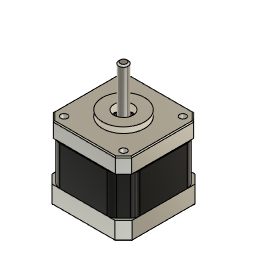
eixo Z 1 v26 (Autodesk Fusion 360 archive; units mm, degrees)
design "motor-17hs4401"
Autodesk Fusion 360 part; units mm, degrees
sketch "Sketch1" plane through (0, 0, 0) normal (0, 0, 1) x (1, 0, 0)
  line L0 (4.1049, 0.5798) -> (36.8951, 0.5798)
  line L1 (41.425, 5.1097) -> (41.425, 37.8999)
  line L2 (36.8951, 42.4298) -> (4.1049, 42.4298)
  line L3 (-0.425, 37.8999) -> (-0.425, 5.1097)
  line L4 (-0.425, 37.8999) -> (4.1049, 42.4298)
  line L5 (36.8951, 0.5798) -> (41.425, 5.1097)
  line L6 (-0.425, 5.1097) -> (4.1049, 0.5798)
  line L7 (36.8951, 42.4298) -> (41.425, 37.8999)
  circle A0 centre (20.5, 21.5048) radius 4.425
  circle A1 centre (5, 37.0048) radius 3.1
  line L8 (-0.425, 21.5048) -> (41.425, 21.5048) construction
  line L9 (20.5, 42.4298) -> (20.5, 0.5798) construction
  line L10 (5, 37.0048) -> (36, 37.0048) construction
  line L11 (36, 37.0048) -> (36, 6.0048) construction
  line L12 (36, 6.0048) -> (5, 6.0048) construction
  line L13 (5, 6.0048) -> (5, 37.0048) construction
  circle A2 centre (36, 37.0048) radius 3.1
  circle A3 centre (36, 6.0048) radius 3.1
  circle A4 centre (5, 6.0048) radius 3.1
  dimension "d3" = 45
  dimension "d4" = 45
  dimension "d5" = 41.85
  dimension "d6" = 41.85
  dimension "d7" = 52.7786
  dimension "d8" = 8.85
  dimension "d9" = 6.2
  dimension "d11" = 31
  dimension "d12" = 31
  constraint horizontal L0
  constraint vertical L1
  constraint horizontal L2
  constraint vertical L3
  constraint parallel L4 L5
  constraint equal L4 L5
  constraint parallel L6 L7
  constraint equal L0 L2
  constraint equal L4 L6
  constraint midpoint L3 L8.start
  constraint midpoint L1 L8.end
  constraint midpoint L2 L9.start
  constraint midpoint L0 L9.end
  constraint coincident A0.centre L9
  constraint coincident A0.centre L8
  constraint horizontal L10
  constraint vertical L11
  constraint horizontal L12
  constraint vertical L13
  constraint coincident A1.centre L10.start
  constraint coincident L10.end L11.start
  constraint coincident L11.end L12.start
  constraint coincident L12.end L13.start
  constraint equal A3 A4
  constraint equal A2 A3
  constraint equal A1 A2
  constraint symmetric L8 L10 L12
  measures "d3" angle of L3 L4
  measures "d4" angle of L0 L6
  measures "d5" distance of L0 L2
  measures "d6" distance of L1 L3
  measures "d7" distance of L4 L5
  measures "d8" diameter of A0
  measures "d9" diameter of A1
  measures "d11" distance of L10.end L11.end
  measures "d12" distance of L11.end L12.end
extrude "Extrude1" add sketch "Sketch1" along normal blind 9.4 makes body 1
fillet "Fillet1" radius 0.5 8 edges at (20.5, 42.4298, 0) (39.1601, 40.1649, 0) (41.425, 21.5048, 0) (39.1601, 2.8448, 0) (20.5, 0.5798, 0) (1.8399, 2.8448, 0) (1.8399, 40.1649, 0) (-0.425, 21.5048, 0) on bodies 1
sketch "Sketch2" plane through (0, 0, 9.4) normal (0, 0, 1) x (-1, 0, 0)
  circle A0 centre (-20.5, -21.5048) radius 4.425
  circle A1 centre (-36, -37.0048) radius 3.1
  circle A2 centre (-5, -37.0048) radius 3.1
  circle A3 centre (-5, -6.0048) radius 3.1
  circle A4 centre (-36, -6.0048) radius 3.1
  line L0 (0.425, -37.8999) -> (0.425, -5.1097)
  line L1 (0.425, -5.1097) -> (-4.1049, -0.5798)
  line L2 (-4.1049, -0.5798) -> (-36.8951, -0.5798)
  line L3 (-36.8951, -0.5798) -> (-41.425, -5.1097)
  line L4 (-41.425, -5.1097) -> (-41.425, -37.8999)
  line L5 (-41.425, -37.8999) -> (-36.8951, -42.4298)
  line L6 (-36.8951, -42.4298) -> (-4.1049, -42.4298)
  line L7 (-4.1049, -42.4298) -> (0.425, -37.8999)
  circle A5 centre (-20.5, -21.5048) radius 3.75
  circle A6 centre (-20.5, -21.5048) radius 2.25
  dimension "d17" = 7.5
  dimension "d18" = -1.5
  constraint concentric A0 A5
  measures "d17" diameter of A5
extrude "Extrude2" add sketch "Sketch2" against normal blind 3 separate body contours A5 makes body 2
extrude "Extrude3" add sketch "Sketch2" against normal blind 4 contours A6 bodies 2
chamfer "Chamfer1" distance 0.5 angle 45 1 edges at (22.5977, 20.6912, 5.4) on bodies 2
sketch "Sketch3" plane through (0, 0, 9.4) normal (0, 0, 1) x (-1, 0, 0)
  circle A0 centre (-20.5, -21.5048) radius 4.425
  circle A1 centre (-36, -37.0048) radius 3.1
  circle A2 centre (-5, -37.0048) radius 3.1
  circle A3 centre (-5, -6.0048) radius 3.1
  circle A4 centre (-36, -6.0048) radius 3.1
  line L0 (0.425, -37.8999) -> (0.425, -5.1097)
  line L1 (0.425, -5.1097) -> (-4.1049, -0.5798)
  line L2 (-4.1049, -0.5798) -> (-36.8951, -0.5798)
  line L3 (-36.8951, -0.5798) -> (-41.425, -5.1097)
  line L4 (-41.425, -5.1097) -> (-41.425, -37.8999)
  line L5 (-41.425, -37.8999) -> (-36.8951, -42.4298)
  line L6 (-36.8951, -42.4298) -> (-4.1049, -42.4298)
  line L7 (-4.1049, -42.4298) -> (0.425, -37.8999)
  line L8 (-8.4787, -31.5261) -> (-8.4787, -11.4835)
  line L9 (-10.4787, -9.4835) -> (-30.5213, -9.4835)
  line L10 (-32.5213, -11.4835) -> (-32.5213, -31.5261)
  line L11 (-30.5213, -33.5261) -> (-10.4787, -33.5261)
  line L12 (-10.4787, -33.5261) -> (-8.4787, -31.5261)
  line L13 (-8.4787, -11.4835) -> (-10.4787, -9.4835)
  line L14 (-30.5213, -9.4835) -> (-32.5213, -11.4835)
  line L15 (-32.5213, -31.5261) -> (-30.5213, -33.5261)
  point P0 (-8.4787, -33.5261)
  point P1 (-8.4787, -9.4835)
  point P2 (-32.5213, -9.4835)
  point P3 (-32.5213, -33.5261)
  dimension "d25" = 2
  dimension "d26" = 2
  dimension "d27" = 2
  dimension "d28" = 2
  dimension "d29" = 2
  dimension "d30" = 2
  dimension "d31" = 2
  dimension "d32" = 2
  constraint parallel L0 L8
  constraint parallel L2 L9
  constraint parallel L4 L10
  constraint parallel L6 L11
  constraint coincident L11 P0
  constraint coincident L8 P0
  constraint coincident L8 P1
  constraint coincident L9 P1
  constraint coincident L9 P2
  constraint coincident L10 P2
  constraint coincident L10 P3
  constraint coincident L11 P3
  measures "d25" distance of L11.end P0
  measures "d26" distance of L8.start P0
  measures "d27" distance of L8.end P1
  measures "d28" distance of L9.start P1
  measures "d29" distance of L9.end P2
  measures "d30" distance of L10.start P2
  measures "d31" distance of L10.end P3
  measures "d32" distance of L11.start P3
extrude "Extrude4" cut sketch "Sketch3" against normal blind 6 contours L8 L9 L10 L11 L12 L13 L14 L15 bodies 1
sketch "Sketch4" plane through (0, 0, 9.4) normal (0, 0, 1) x (-1, 0, 0)
  circle A0 centre (-20.5, -21.5048) radius 3.75
  circle A1 centre (-20.5, -21.5048) radius 6.5
  circle A2 centre (-20.5, -21.5048) radius 3.9
  dimension "d35" = 13
  dimension "d36" = -2.6
  constraint concentric A0 A1
  measures "d35" diameter of A1
extrude "Extrude5" add sketch "Sketch4" against normal blind 3 separate body contours A1 makes body 3
extrude "Extrude6" add sketch "Sketch2" against normal blind 5.5 contours A1 | A2 | A3 | A4 bodies 1
sketch "Sketch5" plane through (0, 0, 3.9) normal (0, 0, -1) x (1, 0, 0)
  circle A0 centre (36, -6.0048) radius 3.1
  circle A1 centre (36, -6.0048) radius 2.5
  arc A2 (36.5, -4.5048) -> (35.5, -4.5048) centre (36, -4.5048) ccw
  arc A3 (35.5, -7.5048) -> (36.5, -7.5048) centre (36, -7.5048) ccw
  line L0 (36, -7.5048) -> (36, -4.5048) construction
  arc A4 (37.5, -6.5048) -> (37.5, -5.5048) centre (37.5, -6.0048) ccw
  arc A5 (34.5, -5.5048) -> (34.5, -6.5048) centre (34.5, -6.0048) ccw
  line L1 (34.5, -6.0048) -> (37.5, -6.0048) construction
  line L2 (37.5, -5.5048) -> (36.5, -5.5048)
  line L3 (35.5, -5.5048) -> (34.5, -5.5048)
  line L4 (35.5, -4.5048) -> (35.5, -5.5048)
  line L5 (35.5, -6.5048) -> (35.5, -7.5048)
  line L6 (34.5, -6.5048) -> (35.5, -6.5048)
  line L7 (36.5, -6.5048) -> (37.5, -6.5048)
  line L8 (36.5, -7.5048) -> (36.5, -6.5048)
  line L9 (36.5, -5.5048) -> (36.5, -4.5048)
  circle A6 centre (5, -6.0048) radius 2.5
  line L10 (5.5, -5.5048) -> (5.5, -4.5048)
  line L11 (4.5, -4.5048) -> (4.5, -5.5048)
  arc A7 (5.5, -4.5048) -> (4.5, -4.5048) centre (5, -4.5048) ccw
  line L12 (4.5, -5.5048) -> (3.5, -5.5048)
  arc A8 (3.5, -5.5048) -> (3.5, -6.5048) centre (3.5, -6.0048) ccw
  line L13 (3.5, -6.5048) -> (4.5, -6.5048)
  line L14 (4.5, -6.5048) -> (4.5, -7.5048)
  arc A9 (4.5, -7.5048) -> (5.5, -7.5048) centre (5, -7.5048) ccw
  line L15 (5.5, -7.5048) -> (5.5, -6.5048)
  line L16 (5.5, -6.5048) -> (6.5, -6.5048)
  arc A10 (6.5, -6.5048) -> (6.5, -5.5048) centre (6.5, -6.0048) ccw
  line L17 (6.5, -5.5048) -> (5.5, -5.5048)
  circle A11 centre (36, -37.0048) radius 2.5
  line L18 (36.5, -36.5048) -> (36.5, -35.5048)
  line L19 (35.5, -35.5048) -> (35.5, -36.5048)
  arc A12 (36.5, -35.5048) -> (35.5, -35.5048) centre (36, -35.5048) ccw
  line L20 (35.5, -36.5048) -> (34.5, -36.5048)
  arc A13 (34.5, -36.5048) -> (34.5, -37.5048) centre (34.5, -37.0048) ccw
  line L21 (34.5, -37.5048) -> (35.5, -37.5048)
  line L22 (35.5, -37.5048) -> (35.5, -38.5048)
  arc A14 (35.5, -38.5048) -> (36.5, -38.5048) centre (36, -38.5048) ccw
  line L23 (36.5, -38.5048) -> (36.5, -37.5048)
  line L24 (36.5, -37.5048) -> (37.5, -37.5048)
  arc A15 (37.5, -37.5048) -> (37.5, -36.5048) centre (37.5, -37.0048) ccw
  line L25 (37.5, -36.5048) -> (36.5, -36.5048)
  circle A16 centre (5, -37.0048) radius 2.5
  line L26 (5.5, -36.5048) -> (5.5, -35.5048)
  line L27 (4.5, -35.5048) -> (4.5, -36.5048)
  arc A17 (5.5, -35.5048) -> (4.5, -35.5048) centre (5, -35.5048) ccw
  line L28 (4.5, -36.5048) -> (3.5, -36.5048)
  arc A18 (3.5, -36.5048) -> (3.5, -37.5048) centre (3.5, -37.0048) ccw
  line L29 (3.5, -37.5048) -> (4.5, -37.5048)
  line L30 (4.5, -37.5048) -> (4.5, -38.5048)
  arc A19 (4.5, -38.5048) -> (5.5, -38.5048) centre (5, -38.5048) ccw
  line L31 (5.5, -38.5048) -> (5.5, -37.5048)
  line L32 (5.5, -37.5048) -> (6.5, -37.5048)
  arc A20 (6.5, -37.5048) -> (6.5, -36.5048) centre (6.5, -37.0048) ccw
  line L33 (6.5, -36.5048) -> (5.5, -36.5048)
  point P0 (36, -6.0048)
  point P1 (36, -6.0048)
  dimension "d41" = 5
  dimension "d42" = 1
  dimension "d43" = 1
  dimension "d44" = 3
  dimension "d45" = 3
  dimension "d48" = -31
  dimension "d49" = -31
  constraint concentric A0 A1
  constraint tangent A2 L8
  constraint tangent A2 L4
  constraint parallel L4 L8
  constraint tangent A3 L4
  constraint tangent A3 L8
  constraint vertical L0
  constraint coincident P1 P0
  constraint midpoint L0 P1
  constraint tangent A4 L6
  constraint tangent A4 L2
  constraint parallel L2 L6
  constraint tangent A5 L2
  constraint tangent A5 L6
  constraint perpendicular L0 L1
  constraint midpoint L1 P1
  constraint collinear L2 L3
  constraint collinear L4 L5
  constraint collinear L6 L7
  constraint collinear L8 L9
  measures "d41" diameter of A1
  measures "d42" distance of L2 L6
  measures "d43" distance of L4 L8
  measures "d44" distance of A3.centre A2.centre
  measures "d45" distance of A5.centre A4.centre
extrude "Extrude7" add sketch "Sketch5" along normal blind 3.6 contours A1 | A6 | A11 | A16 bodies 1
fillet "Fillet2" radius 1 1 edges at (33.6692, 6.9089, 0.3) on bodies 1
fillet "Fillet3" radius 1 1 edges at (2.6692, 6.9089, 0.3) on bodies 1
fillet "Fillet4" radius 1 2 edges at (33.6692, 37.9089, 0.3) (2.6692, 37.9089, 0.3) on bodies 1
sketch "Sketch6" plane through (0, 0, 0) normal (0, 0, -1) x (1, 0, 0)
  circle A0 centre (36, -6.0048) radius 3.1
  circle A1 centre (5, -6.0048) radius 3.1
  circle A2 centre (5, -37.0048) radius 3.1
  circle A3 centre (36, -37.0048) radius 3.1
  circle A4 centre (20.5, -21.5048) radius 4.425
  line L0 (0.075, -5.3168) -> (0.075, -37.6928)
  line L1 (0.075, -37.6928) -> (4.312, -41.9298)
  line L2 (4.312, -41.9298) -> (36.688, -41.9298)
  line L3 (36.688, -41.9298) -> (40.925, -37.6928)
  line L4 (40.925, -37.6928) -> (40.925, -5.3168)
  line L5 (40.925, -5.3168) -> (36.688, -1.0798)
  line L6 (36.688, -1.0798) -> (4.312, -1.0798)
  line L7 (4.312, -1.0798) -> (0.075, -5.3168)
  line L8 (12.25, -41.9298) -> (28.75, -41.9298)
  line L9 (28.75, -41.9298) -> (28.75, -46.5798)
  line L10 (28.75, -46.5798) -> (12.25, -46.5798)
  line L11 (12.25, -46.5798) -> (12.25, -41.9298)
  line L12 (20.5, -21.5048) -> (20.5, -41.9298) construction
  line L13 (36.8951, -0.5798) -> (4.1049, -0.5798)
  dimension "d58" = 16.5
  dimension "d59" = 46
  constraint horizontal L8
  constraint vertical L9
  constraint horizontal L10
  constraint vertical L11
  constraint coincident L2 L8.start
  constraint coincident A4.centre L12.start
  constraint midpoint L2 L12.end
  constraint symmetric L8.start L8.end L12
  measures "d58" distance of L9.end L10.end
  measures "d59" distance of L10 L13
extrude "Extrude8" add sketch "Sketch6" against normal blind 2.8 contours L2 L8 L9 L10 L11 bodies 1
fillet "Fillet5" radius 0.5 3 edges at (12.25, 44.2548, 0) (20.5, 46.5798, 0) (28.75, 44.2548, 0) on bodies 1
sketch "Sketch7" plane through (0, 42.4298, 0) normal (0, 1, 0) x (-1, 0, 0)
  line L0 (-12.25, 2.8) -> (-12.25, 0.5)
  line L1 (-12.25, 0.5) -> (-4.1049, 0.5)
  line L2 (-4.1049, 0.5) -> (-4.1049, 9.4)
  line L3 (-4.1049, 9.4) -> (-36.8951, 9.4)
  line L4 (-36.8951, 9.4) -> (-36.8951, 0.5)
  line L5 (-36.8951, 0.5) -> (-28.75, 0.5)
  line L6 (-28.75, 0.5) -> (-28.75, 2.8)
  line L7 (-28.75, 2.8) -> (-12.25, 2.8)
  line L8 (-28.75, 2.8) -> (-12.25, 2.8)
  line L9 (-12.25, 2.8) -> (-12.25, 9.4)
  line L10 (-12.25, 9.4) -> (-28.75, 9.4)
  line L11 (-28.75, 9.4) -> (-28.75, 2.8)
  line L12 (-12.25, 0.5) -> (-12.25, 2.8)
  constraint horizontal L8
  constraint vertical L9
  constraint horizontal L10
  constraint vertical L11
  constraint coincident L3 L9.end
  constraint coincident L6.end L7.start
  constraint collinear L9 L12
extrude "Extrude9" cut sketch "Sketch7" against normal blind 9 contours L3 L7 L8 L9 L10 L11 bodies 1
sketch "Sketch8" plane through (0, 0, 2.8) normal (0, 0, 1) x (-1, 0, 0)
  line L0 (-28.75, -42.4298) -> (-28.75, -46.5798)
  line L1 (-28.75, -46.5798) -> (-12.25, -46.5798)
  line L2 (-12.25, -46.5798) -> (-12.25, -42.4298)
  line L3 (-12.25, -42.4298) -> (-12.25, -33.4298)
  line L4 (-12.25, -33.4298) -> (-28.75, -33.4298)
  line L5 (-28.75, -33.4298) -> (-28.75, -42.4298)
  line L6 (-13.55, -45.5798) -> (-27.45, -45.5798)
  line L7 (-27.45, -45.5798) -> (-27.45, -33.4298)
  line L8 (-27.45, -33.4298) -> (-13.55, -33.4298)
  line L9 (-13.55, -33.4298) -> (-13.55, -45.5798)
  dimension "d66" = 1.3
  dimension "d67" = 1.3
  dimension "d68" = 1
  constraint horizontal L6
  constraint vertical L7
  constraint horizontal L8
  constraint vertical L9
  constraint coincident L4 L7.end
  measures "d66" distance of L2 L9
  measures "d67" distance of L0 L7
  measures "d68" distance of L1 L6
extrude "Extrude10" add sketch "Sketch8" along normal blind 1 contours L4 L6 L7 L8 L9 bodies 1
sketch "Sketch9" plane through (0, 0, 3.8) normal (0, 0, 1) x (-1, 0, 0)
  line L0 (-13.55, -33.4298) -> (-27.45, -33.4298)
  line L1 (-27.45, -33.4298) -> (-27.45, -45.5798)
  line L2 (-27.45, -45.5798) -> (-13.55, -45.5798) construction
  line L3 (-13.55, -45.5798) -> (-13.55, -33.4298) construction
  line L4 (-12.9, -33.4298) -> (-28.1, -33.4298)
  line L5 (-28.1, -33.4298) -> (-28.1, -45.3421)
  line L6 (-28.1, -45.3421) -> (-12.9, -45.3421)
  line L7 (-12.9, -45.3421) -> (-12.9, -33.4298)
  line L8 (-28.75, -42.4298) -> (-28.75, -46.5798)
  line L9 (-12.9, -45.3421) -> (-12.25, -45.3421) construction
  line L10 (-28.1, -45.3421) -> (-28.75, -45.3421) construction
  line L11 (-12.25, -46.5798) -> (-12.25, -42.4298)
  line L12 (-13.6, -45.3421) -> (-13.6, -34.1298)
  line L13 (-13.6, -34.1298) -> (-27.4, -34.1298)
  line L14 (-27.4, -34.1298) -> (-27.4, -45.3421)
  dimension "d71" = 15.2
  dimension "d75" = -0.7
  constraint horizontal L4
  constraint vertical L5
  constraint horizontal L6
  constraint vertical L7
  constraint perpendicular L7 L9
  constraint coincident L8 L10.end
  constraint perpendicular L8 L10
  constraint coincident L9.end L11
  constraint equal L9 L10
  constraint collinear L0 L4
  measures "d71" distance of L5 L7
extrude "Extrude12" add sketch "Sketch9" along normal blind 5.5 contours L0 L1 L4 L6 L7 L12 L13 L14 | L1 L4 L5 L6 bodies 1
extrude "Extrude13" add sketch "Sketch9" along normal blind 1 contours L6 L12 L13 L14 bodies 1
sketch "Sketch10" plane through (0, 34.1298, 0) normal (0, 1, 0) x (-1, 0, 0)
  line L0 (-27.4, 4.8) -> (-13.6, 4.8)
  line L1 (-13.6, 4.8) -> (-13.6, 9.3)
  line L2 (-13.6, 9.3) -> (-27.4, 9.3)
  line L3 (-27.4, 9.3) -> (-27.4, 4.8)
  line L4 (-27, 9.3) -> (-14, 9.3)
  line L5 (-14, 9.3) -> (-14, 5)
  line L6 (-14, 5) -> (-27, 5)
  line L7 (-27, 5) -> (-27, 9.3)
  line L8 (-27.4, 4.8) -> (-27.4, 9.3)
  line L9 (-13.6, 4.8) -> (-13.6, 9.3)
  line L10 (-15, 9.3) -> (-15, 6)
  line L11 (-15, 6) -> (-26, 6)
  line L12 (-26, 6) -> (-26, 9.3)
  line L13 (-25, 8) -> (-24, 8)
  line L14 (-24, 8) -> (-24, 7)
  line L15 (-24, 7) -> (-25, 7)
  line L16 (-25, 7) -> (-25, 8)
  line L17 (-22.4, 8) -> (-22.4, 7)
  line L18 (-23.4, 8) -> (-22.4, 8)
  line L19 (-23.4, 7) -> (-23.4, 8)
  line L20 (-22.4, 7) -> (-23.4, 7)
  line L21 (-20.8, 8) -> (-20.8, 7)
  line L22 (-21.8, 8) -> (-20.8, 8)
  line L23 (-21.8, 7) -> (-21.8, 8)
  line L24 (-20.8, 7) -> (-21.8, 7)
  line L25 (-19.2, 8) -> (-19.2, 7)
  line L26 (-20.2, 8) -> (-19.2, 8)
  line L27 (-20.2, 7) -> (-20.2, 8)
  line L28 (-19.2, 7) -> (-20.2, 7)
  line L29 (-17.6, 8) -> (-17.6, 7)
  line L30 (-18.6, 8) -> (-17.6, 8)
  line L31 (-18.6, 7) -> (-18.6, 8)
  line L32 (-17.6, 7) -> (-18.6, 7)
  line L33 (-16, 8) -> (-16, 7)
  line L34 (-17, 8) -> (-16, 8)
  line L35 (-17, 7) -> (-17, 8)
  line L36 (-16, 7) -> (-17, 7)
  dimension "d82" = 0.4
  dimension "d83" = 0.4
  dimension "d85" = 0.2
  dimension "d87" = 1
  dimension "d88" = 1
  dimension "d89" = 1
  dimension "d90" = 1
  dimension "d91" = 1
  dimension "d92" = 1
  dimension "d93" = 1
  dimension "d96" = 8
  dimension "d97" = 0
  constraint horizontal L4
  constraint vertical L5
  constraint horizontal L6
  constraint vertical L7
  constraint collinear L2 L4
  constraint parallel L5 L10
  constraint parallel L6 L11
  constraint parallel L7 L12
  constraint coincident L4 L12.end
  constraint coincident L4 L10.start
  constraint horizontal L13
  constraint vertical L14
  constraint horizontal L15
  constraint vertical L16
  measures "d82" distance of L7 L8
  measures "d83" distance of L5 L9
  measures "d85" distance of L0 L6
  measures "d87" distance of L7 L12
  measures "d88" distance of L5 L10
  measures "d89" distance of L6 L11
  measures "d90" distance of L13.start L13.end
  measures "d91" distance of L13.end L14.end
  measures "d92" distance of L12 L16
  measures "d93" distance of L11 L15
extrude "Extrude14" add sketch "Sketch10" along normal blind 13 contours L2 L4 L5 L6 L7 L10 L11 L12 bodies 1
extrude "Extrude15" add sketch "Sketch10" along normal blind 12 contours L13 L14 L15 L16 | L17 L18 L19 L20 | L21 L22 L23 L24 | L25 L26 L27 L28 | L29 L30 L31 L32 | L33 L34 L35 L36 bodies 1
sketch "Sketch11" plane through (0, 0, 9.4) normal (0, 0, 1) x (-1, 0, 0)
  line L0 (-28.75, -42.4298) -> (-28.75, -33.5261)
  line L1 (-28.75, -33.5261) -> (-30.5213, -33.5261)
  line L2 (-30.5213, -33.5261) -> (-32.5213, -31.5261)
  line L3 (-32.5213, -31.5261) -> (-32.5213, -11.4835)
  line L4 (-32.5213, -11.4835) -> (-30.5213, -9.4835)
  line L5 (-30.5213, -9.4835) -> (-10.4787, -9.4835)
  line L6 (-10.4787, -9.4835) -> (-8.4787, -11.4835)
  line L7 (-8.4787, -11.4835) -> (-8.4787, -31.5261)
  line L8 (-8.4787, -31.5261) -> (-10.4787, -33.5261)
  line L9 (-10.4787, -33.5261) -> (-12.25, -33.5261)
  line L10 (-12.25, -33.5261) -> (-12.25, -42.4298)
  line L11 (-12.25, -42.4298) -> (-4.1049, -42.4298)
  line L12 (-4.1049, -42.4298) -> (0.425, -37.8999)
  line L13 (0.425, -37.8999) -> (0.425, -5.1097)
  line L14 (0.425, -5.1097) -> (-4.1049, -0.5798)
  line L15 (-4.1049, -0.5798) -> (-36.8951, -0.5798)
  line L16 (-36.8951, -0.5798) -> (-41.425, -5.1097)
  line L17 (-41.425, -5.1097) -> (-41.425, -37.8999)
  line L18 (-41.425, -37.8999) -> (-36.8951, -42.4298)
  line L19 (-36.8951, -42.4298) -> (-28.75, -42.4298)
  line L20 (-8.1461, -42.4298) -> (-32.8539, -42.4298)
  line L21 (-41.425, -33.8587) -> (-41.425, -9.1509)
  line L22 (-32.8539, -0.5798) -> (-8.1461, -0.5798)
  line L23 (0.425, -7.0798) -> (0.425, -33.8587)
  line L24 (-4.6105, -40.9654) -> (-1.0395, -37.3943)
  line L25 (-4.6105, -2.0443) -> (0.425, -7.0798)
  line L26 (-36.3895, -2.0443) -> (-39.9605, -5.6154)
  line L27 (-36.3895, -40.9654) -> (-39.9605, -37.3943)
  arc A0 (-1.0395, -37.3943) -> (0.425, -33.8587) centre (-4.575, -33.8587) ccw
  arc A1 (-8.1461, -42.4298) -> (-4.6105, -40.9654) centre (-8.1461, -37.4298) ccw
  arc A2 (-36.3895, -40.9654) -> (-32.8539, -42.4298) centre (-32.8539, -37.4298) ccw
  arc A3 (-41.425, -33.8587) -> (-39.9605, -37.3943) centre (-36.425, -33.8587) ccw
  arc A4 (-39.9605, -5.6154) -> (-41.425, -9.1509) centre (-36.425, -9.1509) ccw
  arc A5 (-32.8539, -0.5798) -> (-36.3895, -2.0443) centre (-32.8539, -5.5798) ccw
  arc A6 (-4.6105, -2.0443) -> (-8.1461, -0.5798) centre (-8.1461, -5.5798) ccw
  point P0 (-6.075, -42.4298)
  point P1 (0.425, -35.9298)
  point P2 (0.425, -42.4298)
  point P3 (-6.075, -0.5798)
  point P4 (0.425, -0.5798)
  point P5 (-34.925, -0.5798)
  point P6 (-41.425, -7.0798)
  point P7 (-41.425, -0.5798)
  point P8 (-34.925, -42.4298)
  point P9 (-41.425, -35.9298)
  point P10 (-41.425, -42.4298)
  dimension "d102" = 6.5
  dimension "d103" = 6.5
  dimension "d104" = 6.5
  dimension "d105" = 6.5
  dimension "d106" = 6.5
  dimension "d107" = 6.5
  dimension "d108" = 6.5
  dimension "d109" = 6.5
  dimension "d110" = 5
  constraint horizontal L20
  constraint vertical L21
  constraint horizontal L22
  constraint vertical L23
  constraint collinear L17 L21
  constraint collinear L15 L22
  constraint collinear L13 L23
  constraint collinear L19 L20
  constraint coincident L20 P2
  constraint coincident L23 P2
  constraint coincident L22 P4
  constraint coincident L23 P4
  constraint coincident L22 P7
  constraint coincident L21 P7
  constraint coincident L20 P10
  constraint coincident L21 P10
  constraint coincident P1 L24
  constraint coincident L23 P1
  constraint tangent L24 A0
  constraint tangent L23 A0
  constraint coincident P0 L24
  constraint coincident L20 P0
  constraint tangent L24 A1
  constraint tangent L20 A1
  constraint equal A0 A1
  constraint coincident L20 P8
  constraint coincident P8 L27
  constraint tangent L20 A2
  constraint tangent L27 A2
  constraint equal A0 A2
  constraint coincident P9 L27
  constraint coincident L21 P9
  constraint tangent L27 A3
  constraint tangent L21 A3
  constraint equal A0 A3
  constraint coincident P6 L26
  constraint coincident L21 P6
  constraint tangent L26 A4
  constraint tangent L21 A4
  constraint equal A0 A4
  constraint coincident L22 P5
  constraint coincident P5 L26
  constraint tangent L22 A5
  constraint tangent L26 A5
  constraint equal A0 A5
  constraint coincident P3 L25
  constraint coincident L22 P3
  constraint tangent L25 A6
  constraint tangent L22 A6
  constraint equal A0 A6
  measures "d102" distance of P0 P2
  measures "d103" distance of P1 P2
  measures "d104" distance of P3 P4
  measures "d105" distance of L23.start P4
  measures "d106" distance of P5 P7
  measures "d107" distance of P6 P7
  measures "d108" distance of P8 P10
  measures "d109" distance of P9 P10
  measures "d110" radius of A0
extrude "Extrude16" add sketch "Sketch11" along normal blind 20.5 separate body contours L0 L1 L2 L3 L4 L5 L6 L7 L8 L9 L10 L11 L13 L15 L17 L19 L20 L21 L22 L23 L24 L25 L26 L27 A0 A1 A2 A3 A4 A5 A6 | L0 L1 L2 L3 L4 L5 L6 L7 L8 L9 L10 L20 makes body 4
sketch "Sketch12" plane through (0, 0, 29.9) normal (0, 0, 1) x (-1, 0, 0)
  line L0 (0.425, -7.0798) -> (-4.6105, -2.0443)
  arc A0 (-4.6105, -2.0443) -> (-8.1461, -0.5798) centre (-8.1461, -5.5798) ccw
  line L1 (-8.1461, -0.5798) -> (-32.8539, -0.5798)
  arc A1 (-32.8539, -0.5798) -> (-36.3895, -2.0443) centre (-32.8539, -5.5798) ccw
  line L2 (-36.3895, -2.0443) -> (-39.9605, -5.6154)
  arc A2 (-39.9605, -5.6154) -> (-41.425, -9.1509) centre (-36.425, -9.1509) ccw
  line L3 (-41.425, -9.1509) -> (-41.425, -33.8587)
  arc A3 (-41.425, -33.8587) -> (-39.9605, -37.3943) centre (-36.425, -33.8587) ccw
  line L4 (-39.9605, -37.3943) -> (-36.3895, -40.9654)
  arc A4 (-36.3895, -40.9654) -> (-32.8539, -42.4298) centre (-32.8539, -37.4298) ccw
  line L5 (-32.8539, -42.4298) -> (-8.1461, -42.4298)
  arc A5 (-8.1461, -42.4298) -> (-4.6105, -40.9654) centre (-8.1461, -37.4298) ccw
  line L6 (-4.6105, -40.9654) -> (-1.0395, -37.3943)
  arc A6 (-1.0395, -37.3943) -> (0.425, -33.8587) centre (-4.575, -33.8587) ccw
  line L7 (0.425, -33.8587) -> (0.425, -7.0798)
  line L8 (-36.688, -41.9298) -> (-40.925, -37.6928)
  line L9 (-40.925, -37.6928) -> (-40.925, -5.3168)
  line L10 (-40.925, -5.3168) -> (-36.688, -1.0798)
  line L11 (-36.688, -1.0798) -> (-4.312, -1.0798)
  line L12 (-4.312, -1.0798) -> (-0.075, -5.3168)
  line L13 (-0.075, -5.3168) -> (-0.075, -37.6928)
  line L14 (-0.075, -37.6928) -> (-4.312, -41.9298)
  circle A7 centre (-20.5, -21.5048) radius 4.425
  circle A8 centre (-36, -37.0048) radius 3.1
  circle A9 centre (-5, -37.0048) radius 3.1
  circle A10 centre (-5, -6.0048) radius 3.1
  circle A11 centre (-36, -6.0048) radius 3.1
  line L15 (-4.312, -41.9298) -> (-36.688, -41.9298)
  circle A12 centre (-5, -37.0048) radius 1.75
  circle A13 centre (-36, -37.0048) radius 1.75
  circle A14 centre (-5, -6.0048) radius 1.75
  circle A15 centre (-36, -6.0048) radius 1.75
  dimension "d114" = 3.5
  dimension "d117" = -31
  dimension "d118" = 31
  constraint coincident L14.end L15.start
  constraint coincident L8.start L15.end
  constraint concentric A9 A12
  measures "d114" diameter of A12
extrude "Extrude17" add sketch "Sketch12" along normal blind 7.85 contours L0 A0 A1 L2 A2 A3 L4 A4 A5 L6 A6 L9 L11 L13 A8 A9 A10 A11 L15 | L0 A0 L11 L12 L13 A10 | L0 A10 | L0 A10 | A5 L6 A6 L13 L14 A9 L15 | L6 A9 | L6 A9 | A1 L2 A2 L9 L10 L11 A11 | A3 L4 A4 L8 L9 A8 L15 | L2 A11 | L2 A11 | L4 A8 | L4 A8 | A7 bodies 4
fillet "Fillet6" radius 0.5 8 edges at (38.8065, 39.8113, 37.75) (20.5, 41.9298, 37.75) (40.925, 21.5048, 37.75) (2.1935, 39.8113, 37.75) (0.075, 21.5048, 37.75) (2.1935, 3.1983, 37.75) (20.5, 1.0798, 37.75) (38.8065, 3.1983, 37.75) on bodies 4
extrude "Extrude18" add sketch "Sketch12" along normal blind 1 contours A12 | A13 | A14 | A15 bodies 4
sketch "Sketch13" plane through (0, 0, 37.75) normal (0, 0, 1) x (-1, 0, 0)
  circle A0 centre (-5, -6.0048) radius 1.75
  circle A1 centre (-36, -37.0048) radius 1.75
  circle A2 centre (-36, -6.0048) radius 1.75
  circle A3 centre (-5, -37.0048) radius 1.75
  line L0 (-0.575, -5.5239) -> (-4.5191, -1.5798)
  line L1 (-4.5191, -1.5798) -> (-36.4809, -1.5798)
  line L2 (-36.4809, -1.5798) -> (-40.425, -5.5239)
  line L3 (-40.425, -5.5239) -> (-40.425, -37.4857)
  line L4 (-40.425, -37.4857) -> (-36.4809, -41.4298)
  line L5 (-36.4809, -41.4298) -> (-4.5191, -41.4298)
  line L6 (-4.5191, -41.4298) -> (-0.575, -37.4857)
  line L7 (-0.575, -37.4857) -> (-0.575, -5.5239)
  line L8 (-0.575, -21.5048) -> (-40.425, -21.5048) construction
  line L9 (-20.5, -41.4298) -> (-20.5, -1.5798) construction
  circle A4 centre (-20.5, -21.5048) radius 11
  dimension "d125" = 22
  constraint midpoint L7 L8.start
  constraint midpoint L3 L8.end
  constraint midpoint L5 L9.start
  constraint midpoint L1 L9.end
  constraint midpoint L8 A4.centre
  measures "d125" diameter of A4
extrude "Extrude19" add sketch "Sketch13" along normal blind 3 contours A4 bodies 4
sketch "Sketch14" plane through (0, 0, 40.75) normal (0, 0, 1) x (-1, 0, 0)
  circle A0 centre (-20.5, -21.5048) radius 11
  circle A1 centre (-20.5, -21.5048) radius 5
  dimension "d128" = 10
  constraint concentric A0 A1
  measures "d128" diameter of A1
extrude "Extrude20" cut sketch "Sketch14" against normal blind 4 contours A1 bodies 4
sketch "Sketch15" plane through (0, 0, 36.75) normal (0, 0, 1) x (-1, 0, 0)
  circle A0 centre (-20.5, -21.5048) radius 5
  circle A1 centre (-20.5, -21.5048) radius 4
  circle A2 centre (-20.5, -21.5048) radius 3
  dimension "d131" = -1
  dimension "d132" = -2
extrude "Extrude21" add sketch "Sketch15" along normal blind 0.5 contours A1 bodies 4
sketch "Sketch16" plane through (0, 0, 36.75) normal (0, 0, 1) x (-1, 0, 0)
  circle A0 centre (-20.5, -21.5048) radius 3
  circle A1 centre (-20.5, -21.5048) radius 2.5
  dimension "d135" = 5
  constraint concentric A0 A1
  measures "d135" diameter of A1
extrude "Extrude22" add sketch "Sketch16" along normal blind 25.7 contours A1 bodies 4
sketch "Sketch17" plane through (0, 0, 62.45) normal (0, 0, 1) x (-1, 0, 0)
  circle A0 centre (-20.5, -21.5048) radius 2.5
  line L0 (-18.0214, -21.8316) -> (-20.7353, -23.9937)
  arc A1 (-18.0214, -21.8316) -> (-20.7353, -23.9937) centre (-20.5, -21.5048) ccw
  dimension "d138" = 1.8
  constraint concentric A0 A1
  measures "d138" distance of A0.centre L0
extrude "Extrude23" cut sketch "Sketch17" against normal blind 18 contours A0 L0 bodies 4
chamfer "Chamfer2" distance 0.8 angle 45 1 edges at (22.0578, 19.5495, 62.45) on bodies 4
sketch "Sketch18" plane through (0, 0, 0) normal (0, 0, -1) x (1, 0, 0)
  line L0 (4.312, -41.9298) -> (12.75, -41.9298)
  line L1 (12.75, -41.9298) -> (12.75, -46.0798)
  line L2 (12.75, -46.0798) -> (28.25, -46.0798)
  line L3 (28.25, -46.0798) -> (28.25, -41.9298)
  line L4 (28.25, -41.9298) -> (36.688, -41.9298)
  line L5 (36.688, -41.9298) -> (40.925, -37.6928)
  line L6 (40.925, -37.6928) -> (40.925, -5.3168)
  line L7 (40.925, -5.3168) -> (36.688, -1.0798)
  line L8 (36.688, -1.0798) -> (4.312, -1.0798)
  line L9 (4.312, -1.0798) -> (0.075, -5.3168)
  line L10 (0.075, -5.3168) -> (0.075, -37.6928)
  line L11 (0.075, -37.6928) -> (4.312, -41.9298)
  circle A0 centre (20.5, -21.5048) radius 4.425
  circle A1 centre (36, -37.0048) radius 3.1
  circle A2 centre (5, -37.0048) radius 3.1
  circle A3 centre (5, -6.0048) radius 3.1
  circle A4 centre (36, -6.0048) radius 3.1
  line L12 (6.2591, -10.455) -> (34.9994, -10.8036) construction
  line L13 (34.9994, -10.8036) -> (35.0727, -4.756) construction
  line L14 (35.0727, -4.756) -> (6.3325, -4.4074) construction
  line L15 (6.3325, -4.4074) -> (6.2591, -10.455) construction
  text T0 "-- JSNG --\nStepping Motor\nUS-17HS4401\n" font "Arial" height 2 align centre top in box 28.7424 x 6.0481 at (6.2591, -10.455) x (0.999926, -0.012128) y (0.012128, 0.999926) spacing 1 kerned
extrude "Extrude24" cut sketch "Sketch18" against normal blind 0.5 text T0 bodies 1
copy_body "Body->Comp1" bodies 1 removing the originals makes body 5 in component "Component"
copy_body "Body->Comp2" bodies 2 removing the originals makes body 6 in component "Component'"
copy_body "Body->Comp3" bodies 3 removing the originals makes body 7 in component "Component''"
copy_body "Body->Comp4" bodies 4 removing the originals makes body 8 in component "Component'''"
component "Component" placed x (1, 0, 0) y (0, 1, 0) z (0, 0, 1) at (0, 0, 0)
component "Component'" placed x (1, 0, 0) y (0, 1, 0) z (0, 0, 1) at (0, 0, 0)
component "Component''" placed x (1, 0, 0) y (0, 1, 0) z (0, 0, 1) at (0, 0, 0)
component "Component'''" placed x (1, 0, 0) y (0, 1, 0) z (0, 0, 1) at (0, 0, 0)
equation "d26 = d25"
equation "d28 = d27"
equation "d30 = d29"
equation "d32 = d31"
equation "d103 = d102"
equation "d105 = d104"
equation "d107 = d106"
equation "d109 = d108"
